Autodesk Fusion 360 part; units mm, degrees
(part 2 of 2)
sketch "PinExtraForCapacitive" plane through (0, 0, 7.7) normal (0, 0, 1) x (-1, 0, 0)
  line L0 (-13.048, -42.1183) -> (-7.548, -42.1183)
  arc A0 (-7.548, -45.2183) -> (-7.548, -42.1183) centre (-7.548, -43.6683) ccw
  line L1 (-7.548, -45.2183) -> (-13.048, -45.2183)
  arc A1 (-12.5923, -46.7277) -> (-7.9458, -49.881) centre (-7.9458, -44.881) ccw
  line L2 (-7.9458, -49.881) -> (3.661, -49.881)
  line L3 (3.661, -49.881) -> (3.661, -44.18)
  line L4 (3.661, -44.18) -> (-1, -44.18)
  line L5 (-1, -44.18) -> (-1, 1)
  line L6 (-1, 1) -> (19.542, 1)
  line L7 (19.542, 1) -> (19.542, -44.18)
  line L8 (19.542, -44.18) -> (14.4757, -44.18)
  line L9 (14.4757, -44.18) -> (14.4757, -49.881)
  line L10 (14.4757, -49.881) -> (16.6051, -49.881)
  arc A2 (16.6051, -49.881) -> (21.6051, -44.881) centre (16.6051, -44.881) ccw
  line L11 (21.6051, -44.881) -> (21.6051, 1.7992)
  arc A3 (21.6051, 1.7992) -> (16.6051, 6.7992) centre (16.6051, 1.7992) ccw
  line L12 (16.6051, 6.7992) -> (0.4432, 6.7992)
  arc A4 (0.4432, 6.7992) -> (-9.5568, -3.2008) centre (0.4432, -3.2008) ccw
  line L13 (-10.048, -8.1183) -> (-4.548, -8.1183)
  arc A5 (-4.548, -11.2183) -> (-4.548, -8.1183) centre (-4.548, -9.6683) ccw
  line L14 (-4.548, -11.2183) -> (-9.9659, -11.2183)
  line L15 (-12.048, -12.3683) -> (-6.548, -12.3683)
  arc A6 (-6.548, -15.4683) -> (-6.548, -12.3683) centre (-6.548, -13.9183) ccw
  line L16 (-6.548, -15.4683) -> (-12.025, -15.4683)
  line L17 (-12.025, -15.4683) -> (-12.0907, -15.5174)
  line L18 (-13.048, -16.6183) -> (-7.548, -16.6183)
  arc A7 (-7.548, -19.7183) -> (-7.548, -16.6183) centre (-7.548, -18.1683) ccw
  line L19 (-7.548, -19.7183) -> (-13.048, -19.7183)
  line L20 (-15.048, -20.8683) -> (-9.548, -20.8683)
  arc A8 (-9.548, -23.9683) -> (-9.548, -20.8683) centre (-9.548, -22.4183) ccw
  line L21 (-9.548, -23.9683) -> (-15.048, -23.9683)
  line L22 (-13.048, -25.1183) -> (-7.548, -25.1183)
  arc A9 (-7.548, -28.2183) -> (-7.548, -25.1183) centre (-7.548, -26.6683) ccw
  line L23 (-7.548, -28.2183) -> (-13.048, -28.2183)
  line L24 (-15.048, -29.3683) -> (-9.548, -29.3683)
  arc A10 (-9.548, -32.4683) -> (-9.548, -29.3683) centre (-9.548, -30.9183) ccw
  line L25 (-9.548, -32.4683) -> (-15.048, -32.4683)
  line L26 (-13.048, -33.6183) -> (-7.548, -33.6183)
  arc A11 (-7.548, -36.7183) -> (-7.548, -33.6183) centre (-7.548, -35.1683) ccw
  line L27 (-7.548, -36.7183) -> (-13.048, -36.7183)
  line L28 (-15.048, -37.8683) -> (-9.548, -37.8683)
  arc A12 (-9.548, -40.9683) -> (-9.548, -37.8683) centre (-9.548, -39.4183) ccw
  line L29 (-9.548, -40.9683) -> (-15.048, -40.9683)
  circle A13 centre (18.3729, -46.6488) radius 1
  circle A14 centre (-4.5445, 0) radius 2.5
  circle A15 centre (18.534, 3.3897) radius 1
  line L30 (-1, -42.3372) -> (-4.242, -42.3372)
  line L31 (-4.242, -42.3372) -> (-4.242, -10.0332)
  line L32 (-4.242, -10.0332) -> (-1, -10.0332)
  line L33 (-1, -10.0332) -> (-1, -42.3372)
  line L34 (-2.621, -42.3372) -> (-2.621, -10.0332) construction
  circle A16 centre (-2.621, -39.156) radius 0.85
  circle A17 centre (-2.621, -36.606) radius 0.85
  circle A18 centre (-2.621, -31.506) radius 0.85
  circle A19 centre (-2.621, -28.956) radius 0.85
  circle A20 centre (-2.621, -26.406) radius 0.85
  circle A21 centre (-2.621, -23.856) radius 0.85
  circle A22 centre (-2.621, -21.306) radius 0.85
  circle A23 centre (-2.621, -18.756) radius 0.85
  circle A24 centre (-2.621, -13.656) radius 0.85
  line L35 (-15.048, -40.9683) -> (-13.048, -42.1183)
  line L36 (-13.048, -45.2183) -> (-12.5923, -46.7277)
  line L37 (-9.5568, -3.2008) -> (-10.048, -8.1183)
  line L38 (-9.9659, -11.2183) -> (-12.048, -12.3683)
  line L39 (-12.0907, -15.5174) -> (-13.048, -16.6183)
  line L40 (-13.048, -19.7183) -> (-15.048, -20.8683)
  line L41 (-15.048, -23.9683) -> (-13.048, -25.1183)
  line L42 (-13.048, -28.2183) -> (-15.048, -29.3683)
  line L43 (-15.048, -32.4683) -> (-13.048, -33.6183)
  line L44 (-13.048, -36.7183) -> (-15.048, -37.8683)
  dimension "d71" = 1.7
  dimension "d74" = 5
  dimension "d75" = 2.55
  constraint horizontal L30
  constraint vertical L31
  constraint horizontal L32
  constraint vertical L33
  constraint coincident L5 L30.start
  constraint midpoint L32 L34.end
  constraint coincident L34 A16.centre
  measures "d71" diameter of A16
extrude "Extrude8" cut sketch "PinExtraForCapacitive" against normal blind 2 contours L5 A5 L30 L31 L32 L33 | A5 L31 L32 bodies 1
extrude "Extrude9" cut sketch "PinExtraForCapacitive" against normal blind 7.7 contours A16 | A17 | A18 | A19 | A20 | A21 | A22 | A23 | A24 bodies 1
extrude "Extrude10" add sketch "Border" along normal blind 7.7 separate body contours L0 L1 L2 A0 A1 A3 A4 A5 A6 A7 A8 A10 A12 L4 A13 A15 A17 A20 A22 A23 A24 A25 A27 A28 A29 A30 L9 L10 L11 L12 L13 L14 L15 L16 L17 L18 | A5 A14 A21 | A6 A22 | A13 A29 | A12 A16 A28 | A11 A15 A27 | A9 A10 A26 makes body 13
extrude "Extrude11" cut sketch "PinExtraForCapacitive" against normal blind 7.7 contours A16 | A17 | A18 | A19 | A20 | A21 | A22 | A23 | A24 bodies 13
extrude "Extrude12" cut sketch "Measure_ArduinoNano" along normal blind 7.7 contours L6 A36 L73 | L6 A36 L73 | L6 A36 L73 | L6 A36 L73 | A2 | A3 | L29 L49 A66 | L29 L49 A66 | L49 A66 | A10 | A11 | A14 L192 | A14 L192 | A15 | A16 | A17 | A20 L63 | A20 L63 | A25 | A30 | A31 | A34 | A49 | A56 | A57 | A60 | A62 | A63 | L87 A68 | L87 A68 | L98 A123 L193 | L98 A123 L193 | L98 A123 L193 | L98 A123 L193 | A78 | A94 | A102 | A103 | A121 | A122 | A132 | A133 | A134 | A136 | A137 | A142 | A143 bodies 13
extrude "Extrude16" cut 1 faces at (-16.1495, 1.1473, 6.5) along direction (0, 0, -1) blind 2 on bodies 1 bodies 1
move_body "Move7" [suppressed]
copy_body "CopyPasteBodies1" [suppressed]
move_body "Move4" [suppressed]
move_body "Move5" [suppressed]
move_body "Move6" [suppressed]
move_body "Move8" [suppressed]
move_body "Move9" [suppressed]
move_body "Move10" [suppressed]
copy_body "CopyPasteBodies2" [suppressed]
move_body "Move11" [suppressed]
move_body "Move12" [suppressed]
extrude "Extrude13" [suppressed]
extrude "Extrude14" [suppressed]
move_body "Move13" [suppressed]
hidden bodies 13
equation "SmallBitSize = 1.7 mm"
equation "HalfSmallBitSize = SmallBitSize / 2"
equation "d13 = HalfSmallBitSize"
equation "d14 = HalfSmallBitSize"
equation "d15 = HalfSmallBitSize"
equation "d16 = HalfSmallBitSize"
equation "d17 = HalfSmallBitSize"
equation "d18 = HalfSmallBitSize"
equation "d19 = HalfSmallBitSize"
equation "d20 = HalfSmallBitSize"
equation "d21 = HalfSmallBitSize"
equation "d22 = -HalfSmallBitSize"
equation "d23 = -HalfSmallBitSize"
equation "d24 = -HalfSmallBitSize"
equation "d25 = -HalfSmallBitSize"
equation "d26 = -HalfSmallBitSize"
equation "d27 = -HalfSmallBitSize"
equation "d28 = -HalfSmallBitSize"
equation "d29 = -HalfSmallBitSize"
equation "d30 = -HalfSmallBitSize"
equation "WoodHeight = 7.7 mm"
equation "d40 = WoodHeight"
equation "PinAvailableLength = 5 mm"
equation "d55 = 1.5 mm + PinAvailableLength - 2 mm"
equation "d56 = WoodHeight"
equation "d61 = WoodHeight - 7 mm"
equation "d71 = SmallBitSize"
equation "d78 = WoodHeight * -1"
equation "d80 = WoodHeight"
equation "d82 = WoodHeight * -1"
equation "d84 = WoodHeight"
equation "d95 = WoodHeight"
equation "hasPinPreSoldered = 2 mm"
equation "d103 = -hasPinPreSoldered"
named bodies: "WoodBoard", "WoodBoard (1)", "BorderAndHoles", "BorderAndHoles (1)", "TestTunnel"
